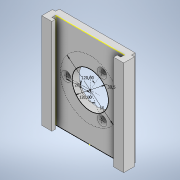
# Autodesk Inventor part: Cycloid_2_base_v2
Saved by Autodesk Inventor 2020.3 (Build 243373000, 373)
## iProperties
Created: 2021-04-22
Part Number: Cycloid_2_base_v2
Material: Generic
Document SubType Name: Modeling
Designer: sanyi
Density: 1 g/cm^3
Appearance: Default
Author: sanyi
Autodesk Inventor part; units mm, degrees
ref_plane "YZ Plane" through (0, 0, 0) normal (1, 0, 0) x (0, 1, 0)
ref_plane "XZ Plane" through (0, 0, 0) normal (0, 1, 0) x (-1, 0, 0)
ref_plane "XY Plane" through (0, 0, 0) normal (0, 0, 1) x (1, 0, 0)
sketch "Sketch2" plane through (0, 0, 0) normal (0, 1, 0) x (-1, 0, 0)
  circle A0 centre (0, 0) radius 15.25
  circle A1 centre (0, 0) radius 25 construction
  circle A2 centre (0, -105) radius 68.1
  line L0 (-85.4561, 0) -> (89.9732, 0) construction
  line L1 (0, 101.2907) -> (0, -205.3562) construction
  circle A3 centre (0, -105) radius 72
  line L2 (53.1573, -36.9) -> (-40.009, -36.9) construction
  line L3 (26.7586, 36.9) -> (26.7586, -36.9)
  line L4 (-26.7586, 36.9) -> (-26.7586, -36.9)
  line L5 (26.7586, -36.9) -> (-26.7586, -36.9)
  line L6 (34.2741, -33.2) -> (-37.5386, -33.2) construction
  line L7 (0, 0) -> (20, 0)
  line L8 (0, 0) -> (-10, 17.3205)
  line L9 (0, 0) -> (-10, -17.3205)
  line L10 (0, 17.3205) -> (-18.0278, 17.3205) construction
  line L11 (0, -17.3205) -> (-18.0278, -17.3205) construction
  circle A4 centre (-10, 17.3205) radius 2.1
  circle A5 centre (20, 0) radius 2.1
  circle A6 centre (-10, -17.3205) radius 2.1
  line L12 (26.7586, 36.9) -> (-26.7586, 36.9)
  dimension "d22" = 30.5
  dimension "d23" = 50
  dimension "d24" = 136.2
  dimension "d25" = 105
  dimension "d26" = 144
  dimension "d40" = 120
  dimension "d41" = 120
  dimension "d42" = 20
  dimension "d43" = 4.2
  constraints: 28 end point, 9 point on line, 7 centre point, 7 coincident, 4 horizontal, 2 equal length, 2 equal radius, 2 parallel, 2 perpendicular, 2 point on circle, 2 tangent, 1 collinear, 1 vertical, 2 other
  measures "d22" diameter of A0
  measures "d23" diameter of A1
  measures "d24" diameter of A2
  measures "d25" distance of point (0, 0) A2.centre
  measures "d26" diameter of A3
  measures "d40" angle of L9 L7
  measures "d41" angle of L8 L9
  measures "d42" distance of L9.start L9.end
  measures "d43" diameter of A4
sketch "Sketch4" plane through (0, 0, 0) normal (0, 1, 0) x (-1, 0, 0)
  line L0 (0, 0) -> (29, 0)
  line L1 (29, 0) -> (29, 3.2)
  line L2 (29, 3.2) -> (26, 3.2)
  line L3 (26, 3.2) -> (26, 6.2)
  line L4 (26, 6.2) -> (34.5, 6.2)
  line L5 (34.5, 6.2) -> (34.5, -2.8)
  line L6 (34.5, -2.8) -> (32, -2.8)
  line L7 (32, -2.8) -> (32, -6)
  line L8 (32, -6) -> (0, -6)
  line L9 (0, -6) -> (0, 0)
  line L10 (0, 0) -> (-29, 0)
  line L11 (-29, 0) -> (-29, 3.2)
  line L12 (-29, 3.2) -> (-26, 3.2)
  line L13 (-26, 3.2) -> (-26, 6.2)
  line L14 (-26, 6.2) -> (-34.5, 6.2)
  line L15 (-34.5, 6.2) -> (-34.5, -2.8)
  line L16 (-34.5, -2.8) -> (-32, -2.8)
  line L17 (-32, -2.8) -> (-32, -6)
  line L18 (-32, -6) -> (0, -6)
  dimension "d44" = 3.2
  dimension "d45" = 3.2
  dimension "d46" = 6
  dimension "d47" = 3
  dimension "d48" = 3
  dimension "d49" = 5.5
  dimension "d50" = 3
  dimension "d51" = 26
  constraints: 38 end point, 9 perpendicular, 8 symmetric about line, 1 horizontal
  measures "d44" distance of L0.end L1.end
  measures "d45" distance of L6.end L7.end
  measures "d46" distance of L8.end L0.start
  measures "d47" distance of L2.end L3.end
  measures "d48" distance between parallel lines of L7 L1
  measures "d49" distance between parallel lines of L5 L1
  measures "d50" distance between parallel lines of L3 L1
  measures "d51" distance between parallel lines of L9 L3
extrude "Extrusion1" add sketch "Sketch4" along normal blind 80
sketch "Sketch6" plane through (-29, 0, 0) normal (0, 0, 1) x (1, 0, 0)
  line L0 (0, 80) -> (58, 80) projected
  line L1 (0, 0) -> (0, 80) projected
  line L2 (0, 0) -> (58, 0) projected
  line L3 (0, 0) -> (58, 0)
  line L4 (58, 0) -> (58, 80) projected
  line L5 (58, 0) -> (58, 80)
  circle A0 centre (29, 40) radius 25 construction
  line L6 (36.5497, 40) -> (21.3269, 40) construction
  line L7 (29, 31.55) -> (29, 50.9237) construction
  line L8 (29, 40) -> (39, 57.3205) construction
  line L9 (29, 40) -> (9, 40) construction
  line L10 (29, 40) -> (39, 22.6795) construction
  circle A1 centre (29, 40) radius 15.25
  point P0 (29, 0)
  dimension "d54" = 50
  dimension "d56" = 120
  dimension "d57" = 120
  dimension "d58" = 20
  dimension "d59" = 30.5
  constraints: 14 end point, 4 coincident, 3 perpendicular, 2 centre point, 2 equal length, 2 point on line, 1 collinear, 1 parallel, 2 other
  measures "d54" diameter of A0
  measures "d56" angle of L9 L10
  measures "d57" angle of L8 L9
  measures "d58" distance of L8.start L9.end
  measures "d59" diameter of A1
extrude "Extrusion2" cut sketch "Sketch6" against normal up to surface (6 mm away) contours A1
hole "Hole1" at (10, 22.6795, 0) at (-20, 40, 0) at (10, 57.3205, 0) direction (0, 0, -1) diameter 4.2 end through all countersink diameter 8 countersink angle 90
body "Solid1"
